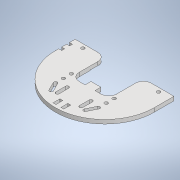
# Autodesk Inventor part: Lift.03.00.00.02
Saved by Autodesk Inventor 2021 (Build 250183000, 183)
## iProperties
Created: 2020-09-20
Part Number: Lift.03.00.00.02
Material: Типовые
Document SubType Name: ЛистМат
Designer: Kostya
Density: 1 g/cm^3
Appearance: По умолчанию
Sheet Metal Rule: По умолчанию_мм
Author: Kostya
Autodesk Inventor part; units mm, degrees
ref_plane "YZ Plane" through (0, 0, 0) normal (1, 0, 0) x (0, 1, 0)
ref_plane "XZ Plane" through (0, 0, 0) normal (0, 1, 0) x (-1, 0, 0)
ref_plane "XY Plane" through (0, 0, 0) normal (0, 0, 1) x (1, 0, 0)
sketch "Эскиз1" plane through (0, 0, 0) normal (0, 1, 0) x (-1, 0, 0)
  line L0 (0, 0) -> (0, -235.2683) construction
  line L1 (250, -250) -> (250, -350)
  line L2 (250, -350) -> (135, -350)
  arc A0 (95, -310) -> (135, -350) centre (135, -310) ccw
  line L3 (95, -310) -> (95, -215)
  arc A1 (95, -215) -> (55, -175) centre (55, -215) ccw
  line L4 (25, -175) -> (25, -205)
  line L5 (25, -205) -> (0, -205)
  line L6 (55, -175) -> (25, -175)
  line L7 (60, -70) -> (60, -120) construction
  line L8 (51.5, -70) -> (51.5, -120)
  line L9 (68.5, -120) -> (68.5, -70)
  arc A2 (68.5, -70) -> (51.5, -70) centre (60, -70) ccw
  arc A3 (51.5, -120) -> (68.5, -120) centre (60, -120) ccw
  line L10 (85.9368, -64.05) -> (108.22, -108.81) construction
  line L11 (93.546, -60.2619) -> (115.8292, -105.0219)
  line L12 (100.6108, -112.5981) -> (78.3276, -67.8381)
  arc A4 (93.546, -60.2619) -> (78.3276, -67.8381) centre (85.9368, -64.05) ccw
  arc A5 (100.6108, -112.5981) -> (115.8292, -105.0219) centre (108.22, -108.81) ccw
  line L13 (12.5, -15) -> (27.43, -15)
  line L14 (27.43, -15) -> (27.43, -50.33)
  line L15 (27.43, -50.33) -> (12.5, -50.33)
  line L16 (12.5, -50.33) -> (12.5, -15)
  circle A6 centre (108.22, -148.81) radius 8.5
  circle A7 centre (108.22, -188.81) radius 8.5
  circle A8 centre (191.91, -330) radius 8.5
  line L17 (-250, -250) -> (-250, -350)
  line L18 (-250, -350) -> (-135, -350)
  arc A9 (-135, -350) -> (-95, -310) centre (-135, -310) ccw
  line L19 (-95, -310) -> (-95, -215)
  arc A10 (-55, -175) -> (-95, -215) centre (-55, -215) ccw
  line L20 (-25, -175) -> (-25, -205)
  line L21 (-25, -205) -> (0, -205)
  line L22 (-55, -175) -> (-25, -175)
  line L23 (-60, -70) -> (-60, -120) construction
  line L24 (-51.5, -70) -> (-51.5, -120)
  line L25 (-68.5, -120) -> (-68.5, -70)
  arc A11 (-51.5, -70) -> (-68.5, -70) centre (-60, -70) ccw
  arc A12 (-68.5, -120) -> (-51.5, -120) centre (-60, -120) ccw
  line L26 (-85.9368, -64.05) -> (-108.22, -108.81) construction
  line L27 (-93.546, -60.2619) -> (-115.8292, -105.0219)
  line L28 (-100.6108, -112.5981) -> (-78.3276, -67.8381)
  arc A13 (-78.3276, -67.8381) -> (-93.546, -60.2619) centre (-85.9368, -64.05) ccw
  arc A14 (-115.8292, -105.0219) -> (-100.6108, -112.5981) centre (-108.22, -108.81) ccw
  line L29 (-12.5, -15) -> (-27.43, -15)
  line L30 (-27.43, -15) -> (-27.43, -50.33)
  line L31 (-27.43, -50.33) -> (-12.5, -50.33)
  line L32 (-12.5, -50.33) -> (-12.5, -15)
  circle A15 centre (-108.22, -148.81) radius 8.5
  circle A16 centre (-108.22, -188.81) radius 8.5
  circle A17 centre (-191.91, -330) radius 8.5
  arc A18 (250, -250) -> (-250, -250) centre (0, -250) ccw
  line L33 (250, -321.45) -> (234.79, -321.45)
  line L34 (234.79, -321.45) -> (234.79, -306.5)
  line L35 (234.79, -306.5) -> (250, -306.5)
  line L36 (250, -281.62) -> (234.79, -281.62)
  line L37 (234.79, -281.62) -> (234.79, -266.67)
  line L38 (234.79, -266.67) -> (250, -266.67)
  line L39 (-250, -321.45) -> (-234.79, -321.45)
  line L40 (-234.79, -321.45) -> (-234.79, -306.5)
  line L41 (-234.79, -306.5) -> (-250, -306.5)
  line L42 (-250, -281.62) -> (-234.79, -281.62)
  line L43 (-234.79, -281.62) -> (-234.79, -266.67)
  line L44 (-234.79, -266.67) -> (-250, -266.67)
  point P0 (60, -95)
  point P1 (97.0784, -86.43)
  point P2 (-60, -95)
  point P3 (-97.0784, -86.43)
  dimension "d2" = 115
  dimension "d4" = 40
  dimension "d5" = 30
  dimension "d7" = 250
  dimension "d9" = 25
  dimension "d10" = 350
  dimension "d11" = 95
  dimension "d12" = 30
  dimension "d13" = 50
  dimension "d14" = 8.5
  dimension "d15" = 64.05
  dimension "d16" = 141.78
  dimension "d17" = 48.22
  dimension "d18" = 70
  dimension "d20" = 241.19
  dimension "d21" = 14.93
  dimension "d22" = 35.33
  dimension "d23" = 12.5
  dimension "d24" = 15
  dimension "d25" = 17
  dimension "d26" = 40
  dimension "d27" = 161.19
  dimension "d28" = 141.78
  dimension "d29" = 20
  dimension "d30" = 58.09
  dimension "d34" = 15.21
  dimension "d35" = 28.55
  dimension "d36" = 14.95
  dimension "d37" = 24.88
  measures "d2" distance of L1.end L2.end
  measures "d4" radius of A1
  measures "d5" distance of L6.start L4.start
  measures "d7" distance between parallel lines of L1 L0
  measures "d9" distance of L4.end L5.end
  measures "d10" distance from line of L0.start L2
  measures "d11" distance of L3.start L3.end
  measures "d12" distance of L4.start L4.end
  measures "d13" distance of L11.start L11.end
  measures "d14" radius of A4
  measures "d15" vertical distance of L0.start L10.start
  measures "d16" distance from line of L1 L10.end
  measures "d17" horizontal distance of L7.end L10.end
  measures "d18" vertical distance of L0.start L7.start
  measures "d20" distance from line of L2 L10.end
  measures "d21" distance of L14.end L15.end
  measures "d22" distance of L13.end L14.end
  measures "d23" distance between parallel lines of L0 L16
  measures "d24" distance from line of L0.start L13
  measures "d25" diameter of A7
  measures "d26" distance of A7.centre A6.centre
  measures "d27" distance from line of L2 A7.centre
  measures "d28" distance from line of L1 A7.centre
  measures "d29" distance from line of L2 A8.centre
  measures "d30" distance from line of L1 A8.centre
  measures "d34" distance between parallel lines of L1 L34
  measures "d35" distance between parallel lines of L2 L33
  measures "d36" distance between parallel lines of L33 L35
  measures "d37" distance between parallel lines of L36 L35
extrude "Пластина1" add sketch "Эскиз1" along normal blind 20 contours L1 L38 L37 L36 L35 L34 L33 L2 A0 L3 A1 L6 L4 L5 L21 L20 L22 A10 L19 A9 L18 L17 L39 L40 L41 L42 L43 L44 A18 | L44 L43 L42 L17 | L41 L40 L39 L17
sketch "Эскиз2" plane through (0, 0, 0) normal (0, -1, 0) x (1, 0, 0)
  arc A0 (100.6108, -112.5981) -> (115.8292, -105.0219) centre (108.22, -108.81) ccw projected
  line L0 (100.6108, -112.5981) -> (78.3276, -67.8381) projected
  arc A1 (93.546, -60.2619) -> (78.3276, -67.8381) centre (85.9368, -64.05) ccw projected
  line L1 (93.546, -60.2619) -> (115.8292, -105.0219) projected
  arc A2 (51.5, -120) -> (68.5, -120) centre (60, -120) ccw projected
  line L2 (51.5, -120) -> (51.5, -70) projected
  arc A3 (68.5, -70) -> (51.5, -70) centre (60, -70) ccw projected
  line L3 (68.5, -70) -> (68.5, -120) projected
  arc A4 (-115.8292, -105.0219) -> (-100.6108, -112.5981) centre (-108.22, -108.81) ccw projected
  line L4 (-115.8292, -105.0219) -> (-93.546, -60.2619) projected
  arc A5 (-78.3276, -67.8381) -> (-93.546, -60.2619) centre (-85.9368, -64.05) ccw projected
  line L5 (-78.3276, -67.8381) -> (-100.6108, -112.5981) projected
  arc A6 (-51.5, -70) -> (-68.5, -70) centre (-60, -70) ccw projected
  line L6 (-51.5, -70) -> (-51.5, -120) projected
  arc A7 (-68.5, -120) -> (-51.5, -120) centre (-60, -120) ccw projected
  line L7 (-68.5, -120) -> (-68.5, -70) projected
  line L8 (12.5, -15) -> (27.43, -15) projected
  line L9 (27.43, -15) -> (27.43, -50.33) projected
  line L10 (27.43, -50.33) -> (12.5, -50.33) projected
  line L11 (12.5, -50.33) -> (12.5, -15) projected
  line L12 (-27.43, -50.33) -> (-27.43, -15) projected
  line L13 (-27.43, -15) -> (-12.5, -15) projected
  line L14 (-12.5, -15) -> (-12.5, -50.33) projected
  line L15 (-12.5, -50.33) -> (-27.43, -50.33) projected
  circle A8 centre (191.91, -330) radius 8.5 projected
  circle A9 centre (108.22, -188.81) radius 8.5 projected
  circle A10 centre (108.22, -148.81) radius 8.5 projected
  circle A11 centre (-191.91, -330) radius 8.5 projected
  circle A12 centre (-108.22, -188.81) radius 8.5 projected
  circle A13 centre (-108.22, -148.81) radius 8.5 projected
  arc A14 (250, -250) -> (-250, -250) centre (0, -250) ccw projected
  line L16 (-250, -266.67) -> (-250, -250) projected
  line L17 (-234.79, -266.67) -> (-250, -266.67) projected
  line L18 (-234.79, -281.62) -> (-234.79, -266.67) projected
  line L19 (-250, -281.62) -> (-234.79, -281.62) projected
  line L20 (-250, -306.5) -> (-250, -281.62) projected
  line L21 (-234.79, -306.5) -> (-250, -306.5) projected
  line L22 (-234.79, -321.45) -> (-234.79, -306.5) projected
  line L23 (-250, -321.45) -> (-234.79, -321.45) projected
  line L24 (-250, -350) -> (-250, -321.45) projected
  line L25 (-135, -350) -> (-250, -350) projected
  arc A15 (-135, -350) -> (-95, -310) centre (-135, -310) ccw projected
  line L26 (-95, -215) -> (-95, -310) projected
  arc A16 (-55, -175) -> (-95, -215) centre (-55, -215) ccw projected
  line L27 (-25, -175) -> (-55, -175) projected
  line L28 (-25, -205) -> (-25, -175) projected
  line L29 (25, -205) -> (-25, -205) projected
  line L30 (25, -175) -> (25, -205) projected
  line L31 (55, -175) -> (25, -175) projected
  arc A17 (95, -215) -> (55, -175) centre (55, -215) ccw projected
  line L32 (95, -310) -> (95, -215) projected
  arc A18 (95, -310) -> (135, -350) centre (135, -310) ccw projected
  line L33 (250, -350) -> (135, -350) projected
  line L34 (250, -250) -> (250, -350) projected
  line L35 (25, -190) -> (-25, -190)
  line L36 (-25, -190) -> (-25, -140)
  line L37 (-25, -140) -> (25, -140)
  line L38 (25, -140) -> (25, -190)
  line L39 (95, -310) -> (95, -215) projected
  line L40 (95, -271.5) -> (145, -271.5)
  line L41 (145, -271.5) -> (145, -316.5)
  line L42 (145, -316.5) -> (95, -316.5)
  line L43 (95, -316.5) -> (95, -271.5)
  line L44 (-95, -215) -> (-95, -310) projected
  line L45 (-95, -316.5) -> (-145, -316.5)
  line L46 (-145, -316.5) -> (-145, -271.5)
  line L47 (-145, -271.5) -> (-95, -271.5)
  line L48 (-95, -271.5) -> (-95, -316.5)
  point P0 (0, 0)
  point P1 (0, -190)
  point P2 (0, -205)
  dimension "d38" = 50
  dimension "d39" = 45
  dimension "d40" = 33.5
  dimension "d41" = 50
  dimension "d42" = 50
  dimension "d43" = 50
  dimension "d44" = 15
  constraints: 24 end point, 6 parallel, 4 point on line, 3 horizontal, 3 perpendicular, 2 midpoint, 1 vertical alignment
  measures "d38" distance of L41.end L42.end
  measures "d39" distance of L40.end L41.end
  measures "d40" distance between parallel lines of L33 L42
  measures "d41" distance between parallel lines of L48 L46
  measures "d42" distance between parallel lines of L37 L35
  measures "d43" distance between parallel lines of L36 L38
  measures "d44" distance between parallel lines of L35 L29
extrude "Вырез1" cut sketch "Эскиз2" against normal blind 2 contours L42 L43 A18 | A18 L32 L40 L41 L42 | L30 L35 L28 L36 L37 L38 | L45 L46 L47 L26 A15 | A15 L48 L45
equation "\"d33\" = Толщина"
equation "\"Толщина\" = 20"
